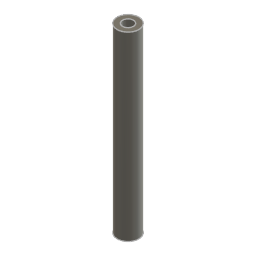
barras 50mm (Autodesk Fusion 360 design; units mm, degrees)
part number: 2026-06-22-13-32-17-644
Autodesk Fusion 360 part; units mm, degrees
sketch "Boceto1" plane through (0, 0, 0) normal (0, 1, 0) x (1, 0, 0)
  circle A0 centre (0, 0) radius 3
  dimension "d1" = 6
  constraint coincident A0.centre origin
  measures "d1" diameter of A0
sketch "Boceto3" plane through (0, 0, 0) normal (0, -1, 0) x (1, 0, 0)
  circle A0 centre (0, 0) radius 3
  circle A1 centre (0, 0) radius 1.525
  dimension "d8" = 3.05
  constraint concentric A0 A1
  measures "d8" diameter of A1
extrude "Extruir2" add sketch "Boceto1" along normal blind 50
sketch "Boceto4" plane through (0, 50, 0) normal (0, 1, 0) x (-1, 0, 0)
  circle A0 centre (0, 0) radius 3
  circle A1 centre (0, 0) radius 1.525
  dimension "d14" = 3.05
  constraint coincident A0.centre A1.centre
  measures "d14" diameter of A1
hole "Agujero3" at (0, 50, 0) direction (0, -1, 0) diameter 3 depth 15 tip angle 118
hole "Agujero4" at (0, 0, 0) direction (0, 1, 0) diameter 3 depth 15 tip angle 118
